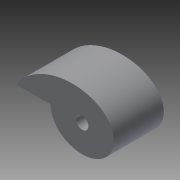
# Autodesk Inventor part: cam 1
Saved by Autodesk Inventor 2014 (Build 180170000, 170)
## iProperties
Created: 2014-05-19
Part Number: cam 1
Material: Generic
Document SubType Name: Modeling
Designer: jyesowitz
Density: 1 g/cm^3
Appearance: Default
Author: jyesowitz
Autodesk Inventor part; units mm, degrees
ref_plane "YZ Plane" through (0, 0, 0) normal (1, 0, 0) x (0, 1, 0)
ref_plane "XZ Plane" through (0, 0, 0) normal (0, 1, 0) x (-1, 0, 0)
ref_plane "XY Plane" through (0, 0, 0) normal (0, 0, 1) x (1, 0, 0)
sketch "Sketch1" plane through (0, 0, 0) normal (0, 0, 1) x (1, 0, 0)
  ellipse E0 centre (0.0127, -0.0088) end of major axis (32.1691, -0.0088) minor radius 27.8638 (-32.1437, -0.0088) -> (30.8279, 7.9544) ccw
  line L0 (30.8279, 7.9544) -> (21.9875, 33.6403) construction
  line L1 (21.9875, 33.6403) -> (-30.3141, 42.418) construction
  line L2 (-30.3141, 42.418) -> (-59.3845, 13.3663) construction
  line L3 (-59.3845, 13.3663) -> (-67.0687, -0.0088) construction
  spline S0 degree 4 poles (30.8279, 7.9544) (21.9875, 33.6403) (-30.3141, 42.418) (-59.3845, 13.3663) (-67.0687, -0.0088) knots 1 1 1 1 1 2 2 2 2 2
  line L4 (-67.0687, -0.0088) -> (-32.1437, -0.0088)
  circle A0 centre (0.0127, -0.0088) radius 6.35
  point P0 (0, 0)
  dimension "d62" = 32.1564
  dimension "d63" = 27.8638
  dimension "d42" = 42.418
  dimension "d43" = 67.0687
  dimension "d44" = 32.1437
  dimension "d45" = 41.0985
  dimension "d46" = 15.4253
  dimension "d47" = 53.0331
  dimension "d48" = 27.1647
  dimension "d53" = 125.491
  dimension "d57" = 7.9544
  dimension "d64" = 12.7
  constraints: 2 end point, 1 centre point, 1 coincident, 1 horizontal, 1 horizontal alignment, 10 other
  measures "d42" vertical distance of point (0, 0) L1.end
  measures "d43" distance of point (0, 0) L3.end
  measures "d44" distance of point (0, 0) L4.end
  measures "d45" distance of L1.end L2.end
  measures "d46" distance of L2.end L3.end
  measures "d47" distance of L0.end L1.end
  measures "d48" distance of L0.start L0.end
  measures "d53" angle of L2 L1
  measures "d57" vertical distance of point (0, 0) L0.start
  measures "d64" diameter of A0
extrude "Extrusion1" add sketch "Sketch1" against normal blind 50.8
body "Solid1"
